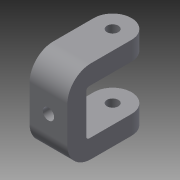
# Autodesk Inventor part: PulleyHolder
Saved by Autodesk Inventor 2015 (Build 190159000, 159)
## iProperties
Created: 2017-01-05
Part Number: PulleyHolder
Material: Generic
Document SubType Name: Modeling
Designer: Ernest
Density: 1 g/cm^3
Appearance: Default
Author: Ernest
Autodesk Inventor part; units mm, degrees
ref_plane "YZ Plane" through (0, 0, 0) normal (1, 0, 0) x (0, 1, 0)
ref_plane "XZ Plane" through (0, 0, 0) normal (0, 1, 0) x (-1, 0, 0)
ref_plane "XY Plane" through (0, 0, 0) normal (0, 0, 1) x (1, 0, 0)
sketch "Sketch1" plane through (0, 0, 0) normal (0, 0, 1) x (1, 0, 0)
  arc A0 (5, 0) -> (-5, 0) centre (0, 0) ccw
  line L0 (-5, -17) -> (5, -17)
  line L1 (5, -17) -> (5, 0)
  line L2 (-5, -17) -> (-5, 0)
  circle A1 centre (0, 0) radius 1.5
  dimension "d0" = 3
  dimension "d1" = 5
  dimension "d2" = 17
  constraints: 6 end point, 2 centre point, 2 coincident, 2 point on circle, 2 tangent, 1 horizontal
  measures "d0" diameter of A1
  measures "d1" radius of A0
  measures "d2" distance from line of L0 point (0, 0)
extrude "Extrusion1" add sketch "Sketch1" along normal blind 22
sketch "Sketch2" plane through (5, -17, 0) normal (1, 0, 0) x (0, 0, -1)
  line L0 (0, 17) -> (0, 17) projected
  line L1 (0, 17) -> (-22, 17) projected
  line L2 (-22, 17) -> (-22, 17) projected
  line L3 (0, 17) -> (-22, 17) projected
  line L4 (0, 0) -> (0, 17) projected
  line L5 (0, 17) -> (-22, 17) projected
  line L6 (-22, 0) -> (-22, 17) projected
  line L7 (0, 0) -> (-22, 0) projected
  line L8 (-17, 5) -> (-5, 5)
  line L9 (-5, 5) -> (-5, 25)
  line L10 (-5, 25) -> (-17, 25)
  line L11 (-17, 25) -> (-17, 5)
  dimension "d5" = 5
  dimension "d6" = 5
  dimension "d7" = 5
  dimension "d8" = 20
  constraints: 8 end point, 2 parallel, 1 horizontal, 1 perpendicular
  measures "d5" distance between parallel lines of L7 L8
  measures "d6" distance between parallel lines of L11 L6
  measures "d7" distance between parallel lines of L4 L9
  measures "d8" distance of L10.end L8.start
extrude "Extrusion2" cut sketch "Sketch2" against normal blind 22 contours L9 L8 L11 L1 | L1 L11 L10 L9
sketch "Sketch3" plane through (-5, -17, 0) normal (0, -1, 0) x (1, 0, 0)
  line L0 (0, 0) -> (10, 0) projected
  line L1 (10, 0) -> (10, 22) projected
  line L2 (0, 22) -> (10, 22) projected
  line L3 (0, 0) -> (0, 22) projected
  circle A0 centre (5, 11) radius 1.5
  point P0 (5, 0)
  dimension "d11" = 22
  dimension "d12" = 10
  dimension "d13" = 3
  dimension "d14" = 5
  dimension "d15" = 11
  constraints: 1 centre point
  measures "d11" distance of L0.start L2.start
  measures "d12" distance of L2.start L1.end
  measures "d13" diameter of A0
  measures "d14" distance from line of L3 A0.centre
  measures "d15" distance from line of L2 A0.centre
extrude "Extrusion3" cut sketch "Sketch3" against normal blind 6 contours A0
fillet "Fillet1" radius 6.25 2 edges at (0, -17, 22) (0, -17, 0)
fillet "Fillet2" radius 0.75 2 edges at (0, -12, 17) (0, -12, 5)
equation "\"d14\" = 0.5 * d12"
equation "\"d15\" = 0.5 * d11"
body "Solid1"
